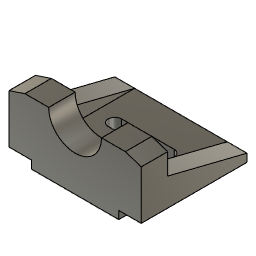
Tutorial Part 13 v2 (Autodesk Fusion 360 design; units mm, degrees)
Autodesk Fusion 360 part; units mm, degrees
note: some values were not read from the file. Chosen so that the rebuilt part matches the saved one: a direction.
sketch "Sketch1" plane through (0, 0, 0) normal (0, 1, 0) x (1, 0, 0)
  line L0 (-33, 47) -> (33, 47)
  line L1 (33, 47) -> (33, 41)
  line L2 (33, 41) -> (50, 41)
  line L3 (50, 41) -> (50, 0)
  line L4 (-50, 0) -> (-50, 41)
  line L5 (-50, 41) -> (-33, 41)
  line L6 (-33, 41) -> (-33, 47)
  arc A0 (20, 0) -> (-20, 0) centre (0, 0) ccw
  line L7 (50, 0) -> (20, 0)
  line L8 (-20, 0) -> (-50, 0)
  line L9 (50, 35) -> (35, 35)
  line L10 (35, 35) -> (35, 20)
  line L11 (35, 20) -> (50, 20)
  line L12 (50, 20) -> (50, 35)
  line L13 (-50, 35) -> (-35, 35)
  line L14 (-35, 35) -> (-35, 20)
  line L15 (-35, 20) -> (-50, 20)
  line L16 (-50, 20) -> (-50, 35)
  line L17 (-50, 35) -> (50, 35)
  dimension "d1" = 100
  dimension "d2" = 47
  dimension "d3" = 17
  dimension "d4" = 6
  dimension "d5" = 40
  dimension "d6" = 50
  dimension "d7" = 15
  dimension "d8" = 15
  dimension "d9" = 6
  constraint horizontal L0
  constraint perpendicular L0 L1
  constraint perpendicular L1 L2
  constraint perpendicular L2 L3
  constraint perpendicular L3 L7
  constraint perpendicular L4 L7
  constraint perpendicular L4 L5
  constraint perpendicular L0 L6
  constraint collinear L2 L5
  constraint equal L2 L5
  constraint coincident A0.end L7
  constraint collinear L7 L8
  constraint coincident A0.centre L7
  constraint coincident A0.centre origin
  constraint horizontal L9
  constraint vertical L10
  constraint horizontal L11
  constraint vertical L12
  constraint coincident L3 L9.start
  constraint horizontal L13
  constraint vertical L14
  constraint horizontal L15
  constraint vertical L16
  constraint coincident L4 L13.start
  constraint collinear L11 L15
  constraint equal L11 L15
  constraint equal L10 L14
  measures "d1" distance of L3.end L4.start
  measures "d2" distance of L0 L7
  measures "d3" distance of L4.end L5.end
  measures "d4" distance of L0.start L5.end
  measures "d5" diameter of A0
  measures "d6" distance of L3 A0.centre
  measures "d7" distance of L9.start L9.end
  measures "d8" distance of L9.end L10.end
  measures "d9" distance of L2 L9
extrude "Extrude1" add sketch "Sketch1" along normal blind 80 contours L0 L1 L2 L3 L4 L5 L6 L9 L13 L17
extrude "Extrude2" add sketch "Sketch1" along normal blind 80 contours L4 L13 L14 L15 L16 L17 | L3 L9 L10 L11 L12 L17
extrude "Extrude3" add sketch "Sketch1" along normal blind 20 contours L3 L4 A0 L7 L8 L10 L11 L14 L15 L17
chamfer "Chamfer1" distance 12 distance2 4 1 edges at (50, 10, 0) measured on face at (40, 6.6667, 0)
chamfer "Chamfer2" distance 4 distance2 12 1 edges at (-50, 10, 0) measured on face at (-50, 33.3333, -34)
chamfer "Chamfer3" distance 15 distance2 60 2 edges at (42.5, 80, -20) (-42.5, 80, -20) measured on face at (45, 80, -32) measured on face at (45, 80, -32)
sketch "Sketch2" plane through (0, 0, -35) normal (0, 0, 1) x (-1, 0, 0)
  line L0 (35, -20) -> (-35, -20)
  line L1 (-35, -20) -> (-35, -80)
  line L2 (-35, -80) -> (35, -80)
  line L3 (35, -80) -> (35, -20)
  line L4 (20, -45) -> (-20, -45)
  arc A0 (-20, -45) -> (-20, -55) centre (-20, -50) ccw
  line L5 (-20, -55) -> (20, -55)
  arc A1 (20, -55) -> (20, -45) centre (20, -50) ccw
  line L6 (25, -50) -> (-25, -50) construction
  line L7 (50, -80) -> (50, -20)
  dimension "d22" = 5
  dimension "d23" = 30
  dimension "d24" = 40
  dimension "d25" = 30
  constraint tangent L4 A0
  constraint tangent A0 L5
  constraint parallel L4 L5
  constraint tangent L5 A1
  constraint tangent L4 A1
  constraint midpoint A1 L6.start
  constraint midpoint A0 L6.end
  constraint perpendicular L1 L6
  measures "d22" radius of A0
  measures "d23" distance of L2 A1.centre
  measures "d24" distance of A0.end L5.end
  measures "d25" distance of A1.centre L7
extrude "Extrude4" cut sketch "Sketch2" against normal through all contours L4 A0 L5 A1
